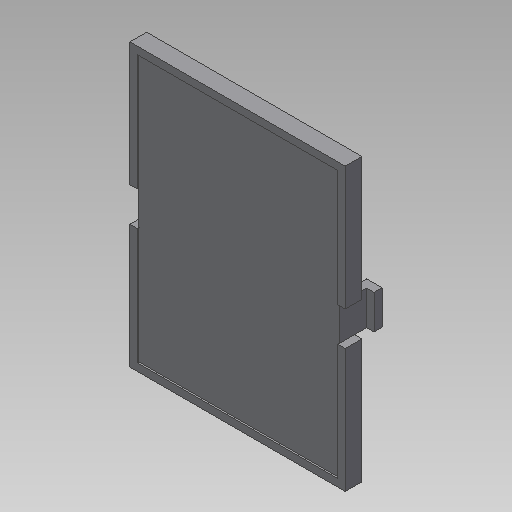
# Autodesk Inventor part: D2MG cover
Saved by Autodesk Inventor 2018 (Build 220112000, 112)
## iProperties
Created: 2015-06-28
Part Number: D2MG cover
Material: Типовые
Document SubType Name: Modeling
Designer: Abbath
Density: 1 g/cm^3
Appearance: По умолчанию
Author: Abbath
Autodesk Inventor part; units mm, degrees
ref_plane "YZ Plane" through (0, 0, 0) normal (1, 0, 0) x (0, 1, 0)
ref_plane "XZ Plane" through (0, 0, 0) normal (0, 1, 0) x (-1, 0, 0)
ref_plane "XY Plane" through (0, 0, 0) normal (0, 0, 1) x (1, 0, 0)
sketch "Эскиз1" plane through (0, 0, 0) normal (0, 0, 1) x (1, 0, 0)
  line L0 (-16.05, 21) -> (16.05, 21)
  line L1 (16.05, 21) -> (16.05, -21)
  line L2 (16.05, -21) -> (-16.05, -21)
  line L3 (-16.05, -21) -> (-16.05, 21)
  point P0 (0, 0)
  point P1 (0, 21)
  point P2 (16.05, 0)
  dimension "d0" = 32.1
  dimension "d1" = 42
  constraints: 8 end point, 2 midpoint, 2 parallel, 1 horizontal, 1 horizontal alignment, 1 perpendicular, 1 vertical alignment
  measures "d0" distance between parallel lines of L1 L3
  measures "d1" distance between parallel lines of L2 L0
extrude "Выдавливание1" add sketch "Эскиз1" along normal blind 2.5
sketch "Эскиз2" plane through (0, 0, 0) normal (0, 1, 0) x (-1, 0, 0)
  line L0 (16.05, 0) -> (-16.05, 0) construction
  line L1 (16.05, 0) -> (16.05, 2.5) construction
  line L2 (-16.05, 2.5) -> (16.05, 2.5) construction
  line L3 (-16.05, 0) -> (-16.05, 2.5) construction
  line L4 (-13.75, 0) -> (-13.75, -3)
  line L5 (-13.75, -3) -> (-16.05, -3)
  line L6 (-16.05, -3) -> (-16.05, -1.8)
  line L7 (-16.05, -1.8) -> (-14.95, -1.8)
  line L8 (-14.95, -1.8) -> (-14.95, 0)
  line L9 (-14.95, 0) -> (-13.75, 0)
  line L10 (13.75, 0) -> (13.75, -3)
  line L11 (13.75, -3) -> (16.05, -3)
  line L12 (16.05, -3) -> (16.05, -1.8)
  line L13 (16.05, -1.8) -> (14.95, -1.8)
  line L14 (14.95, -1.8) -> (14.95, 0)
  line L15 (14.95, 0) -> (13.75, 0)
  point P0 (0, 0)
  dimension "d4" = 2.3
  dimension "d5" = 1.2
  dimension "d6" = 5.5
  constraints: 24 end point, 6 horizontal, 6 vertical, 5 collinear, 4 equal length
  measures "d4" distance between parallel lines of L10 L12
  measures "d5" distance between parallel lines of L8 L4
  measures "d6" distance between parallel lines of L5 L2
extrude "Выдавливание2" add sketch "Эскиз2" along normal mid plane 5.1
sketch "Эскиз3" plane through (0, 0, 2.5) normal (0, 0, 1) x (1, 0, 0)
  line L0 (17.05, 2.55) -> (14.95, 2.55)
  line L1 (14.95, 2.55) -> (14.95, -2.55)
  line L2 (14.95, -2.55) -> (17.05, -2.55)
  line L3 (17.05, -2.55) -> (17.05, 2.55)
  line L4 (-14.95, 2.55) -> (-17.05, 2.55)
  line L5 (-17.05, 2.55) -> (-17.05, -2.55)
  line L6 (-17.05, -2.55) -> (-14.95, -2.55)
  line L7 (-14.95, -2.55) -> (-14.95, 2.55)
  line L8 (-16.05, 21) -> (-16.05, -21) construction
  line L9 (16.05, -21) -> (16.05, 21) construction
  line L10 (16.05, -2.55) -> (16.05, 2.55) construction
  line L11 (14.95, 2.55) -> (16.05, 2.55) construction
  line L12 (14.95, -2.55) -> (14.95, 2.55) construction
  line L13 (16.05, -2.55) -> (14.95, -2.55) construction
  line L14 (-14.95, 2.55) -> (-14.95, -2.55) construction
  line L15 (-16.05, 2.55) -> (-14.95, 2.55) construction
  line L16 (-16.05, 2.55) -> (-16.05, -2.55) construction
  line L17 (-14.95, -2.55) -> (-16.05, -2.55) construction
  point P0 (0, 0)
  dimension "d9" = 1
  dimension "d10" = 1
  constraints: 16 end point, 6 collinear, 4 parallel, 2 horizontal, 2 perpendicular
  measures "d9" distance between parallel lines of L5 L8
  measures "d10" distance between parallel lines of L3 L9
extrude "Выдавливание3" cut sketch "Эскиз3" against normal up to surface (4.3 mm away)
sketch "Эскиз4" plane through (0, 0, 0) normal (0, 0, -1) x (-1, 0, 0)
  line L0 (13.75, -18.7) -> (-13.75, -18.7)
  line L1 (-13.75, -18.7) -> (-13.75, 18.7)
  line L2 (-13.75, 18.7) -> (13.75, 18.7)
  line L3 (13.75, 18.7) -> (13.75, -18.7)
  line L4 (-16.05, -21) -> (16.05, -21) construction
  line L5 (16.05, 21) -> (-16.05, 21) construction
  line L6 (13.75, -2.55) -> (13.75, 2.55) construction
  line L7 (-13.75, 2.55) -> (-13.75, -2.55) construction
  line L8 (16.05, -2.55) -> (16.05, -21) construction
  point P0 (0, 0)
  dimension "d13" = 2.3
  dimension "d14" = 2.3
  dimension "d15" = 2.3
  constraints: 8 end point, 2 collinear, 2 parallel, 1 horizontal, 1 perpendicular
  measures "d13" distance between parallel lines of L8 L3
  measures "d14" distance between parallel lines of L0 L4
  measures "d15" distance between parallel lines of L5 L2
extrude "Выдавливание4" cut sketch "Эскиз4" against normal blind 0.25
sketch "Эскиз5" plane through (0, 0, 2.5) normal (0, 0, 1) x (1, 0, 0)
  line L0 (14.95, 19.9) -> (-14.95, 19.9)
  line L1 (-14.95, 19.9) -> (-14.95, -19.9)
  line L2 (-14.95, -19.9) -> (14.95, -19.9)
  line L3 (14.95, -19.9) -> (14.95, 19.9)
  line L4 (14.95, -2.55) -> (14.95, 2.55) construction
  line L5 (-14.95, 2.55) -> (-14.95, -2.55) construction
  line L6 (16.05, 2.55) -> (16.05, 21) construction
  line L7 (16.05, 21) -> (-16.05, 21) construction
  line L8 (-16.05, -21) -> (16.05, -21) construction
  point P0 (0, 0)
  dimension "d18" = 1.1
  dimension "d19" = 1.1
  dimension "d20" = 1.1
  constraints: 8 end point, 2 collinear, 2 parallel, 1 horizontal, 1 perpendicular
  measures "d18" distance between parallel lines of L3 L6
  measures "d19" distance between parallel lines of L8 L2
  measures "d20" distance between parallel lines of L7 L0
extrude "Выдавливание5" cut sketch "Эскиз5" against normal blind 0.25
equation "\"d14\" = d13"
equation "\"d15\" = d13"
equation "\"d19\" = d18"
equation "\"d20\" = d18"
